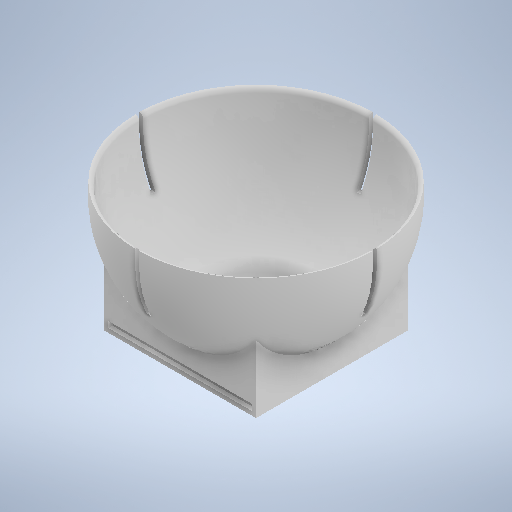
# Autodesk Inventor part: Socket
Saved by Autodesk Inventor 2025 (Build 290162000, 162)
## iProperties
Created: 2024-11-17
Part Number: Socket
Material: Generic
Document SubType Name: Modeling
Designer: ethan
Density: 1 g/cm^3
Appearance: Default
Author: ethan
Autodesk Inventor part; units mm, degrees
ref_plane "YZ Plane" through (0, 0, 0) normal (1, 0, 0) x (0, 1, 0)
sketch "Sketch1" plane through (0, 0, 0) normal (0, 0, 1) x (1, 0, 0)
  circle A0 centre (0, 0) radius 28 construction
  circle A1 centre (0, 0) radius 29 construction
  circle A2 centre (0, 0) radius 28
  circle A3 centre (0, 0) radius 29
  line L0 (0, 0) -> (27.8935, 2.4404)
  line L1 (0, 0) -> (28, 0) construction
  line L2 (0, 0) -> (0, -29.5121)
  line L3 (0, -28) -> (0, -29)
  line L4 (27.8935, 2.4404) -> (28.8971, 2.4404)
  dimension "d0" = 56
  dimension "d1" = 58
  dimension "d2" = 5
  constraints: 10 end point, 4 centre point, 4 coincident, 4 point on circle, 2 concentric, 2 horizontal, 2 point on line, 1 equal length, 1 vertical
  measures "d0" diameter of A0
  measures "d1" diameter of A1
  measures "d2" angle of L1 L0
revolve "Revolution1" add sketch "Sketch1" angle 360 about axis through (0, 0, 0) along (0, -1, 0) picked at (16.0405, -23.5642) contours A2 L4 A3 L2
sketch "Sketch2" plane through (0, 2.4404, 0) normal (0, 1, 0) x (1, 0, 0)
  line L0 (-0.5, -30) -> (0.5, -30)
  line L1 (0.5, -30) -> (0.5, 30)
  line L2 (0.5, 30) -> (-0.5, 30)
  line L3 (-0.5, 30) -> (-0.5, -30)
  line L4 (-0.5, -30) -> (0.5, 30) construction
  line L5 (0.5, -30) -> (-0.5, 30) construction
  line L6 (30, -0.5) -> (-30, -0.5)
  line L7 (-30, -0.5) -> (-30, 0.5)
  line L8 (-30, 0.5) -> (30, 0.5)
  line L9 (30, 0.5) -> (30, -0.5)
  circle A0 centre (0, 0) radius 28.8971 projected
  line L10 (30, -0.5) -> (-30, 0.5) construction
  line L11 (-30, -0.5) -> (30, 0.5) construction
  point P0 (0.5, 0.5)
  point P1 (-0.5, 0.5)
  point P2 (-0.5, -0.5)
  point P3 (0.5, -0.5)
  dimension "d4" = 1
  dimension "d5" = 60
  dimension "d6" = 60
  dimension "d7" = 1
  constraints: 24 end point, 4 midpoint, 4 parallel, 2 horizontal, 2 perpendicular
  measures "d4" distance of L2.end L1.end
  measures "d5" distance of L1.end L0.end
  measures "d6" distance of L7.end L8.end
  measures "d7" distance of L6.end L7.end
extrude "Extrusion1" cut sketch "Sketch2" against normal blind 15 contours L3 A0 L1 L0 | L3 L6 L1 A0 | L6 A0 L8 L3 | L3 L8 L1 L6 | L6 L7 L8 A0 | L1 L8 A0 L6 | A0 L8 L9 L6 | L3 A0 L1 L8 | L3 L2 L1 A0
ref_plane "Work Plane1" through (0, -29, 0) normal (0, 1, 0) x (-1, 0, 0)
sketch "Sketch3" plane through (0, -29, 0) normal (0, 1, 0) x (-1, 0, 0)
  arc A0 (-0.5, 28.8928) -> (-28.8928, 0.5) centre (0, 0) ccw projected
  arc A1 (-0.5, -26.1344) -> (0.5, -26.1344) centre (0, 0) ccw projected
  line L0 (0.5, -25.0201) -> (0.5, -26.1344) projected
  arc A2 (-0.5, -25.0201) -> (0.5, -25.0201) centre (0, 0) ccw projected
  line L1 (-0.5, -26.1344) -> (-0.5, -25.0201) projected
  circle A3 centre (0, 0) radius 26.1392
  line L2 (18.485, 18.4813) -> (-18.485, 18.4813)
  line L3 (-18.485, 18.4813) -> (-18.485, -18.4813)
  line L4 (-18.485, -18.4813) -> (18.485, -18.4813)
  line L5 (18.485, -18.4813) -> (18.485, 18.4813)
  line L6 (18.485, 18.4813) -> (-18.485, -18.4813) construction
  line L7 (-18.485, 18.4813) -> (18.485, -18.4813) construction
  dimension "d11" = 36.97
  constraints: 12 end point, 2 midpoint, 2 parallel, 2 point on circle, 1 centre point, 1 coincident, 1 horizontal, 1 perpendicular
  measures "d11" distance of L4.end L3.end
extrude "Extrusion2" add sketch "Sketch3" along normal up to surface contours L3 L2 L5 L4
sketch "Sketch4" plane through (0, -29, 0) normal (0, -1, 0) x (1, 0, 0)
  circle A0 centre (0, 0) radius 13.5
  dimension "d14" = 27
  constraints: 1 centre point, 1 coincident
  measures "d14" diameter of A0
extrude "Extrusion3" cut sketch "Sketch4" against normal blind 10
fillet "Fillet1" radius 3 1 edges at (-13.5, -24.5306, 0)
fillet "Fillet2" radius 1 4 edges at (-19.7236, 2.4404, 19.7236) (-19.7236, 2.4404, -19.7236) (19.7236, 2.4404, -19.7236) (19.7236, 2.4404, 19.7236)
sketch "Sketch5" plane through (-18.485, -29, 18.4813) normal (0, 0, 1) x (1, 0, 0)
  line L0 (0, 0) -> (0, 16.4404) construction
  line L1 (0, 0) -> (1, 0) construction
  line L2 (1, 0) -> (1, 1) construction
  line L3 (1, 1) -> (0, 1) construction
  line L4 (0, 1) -> (0, 0) construction
  arc A0 (0, 16.4404) -> (36.97, 16.4404) centre (18.485, 29) ccw construction
  line L5 (0, 0) -> (0, 16.4404) construction
  line L6 (0, 0) -> (36.97, 0) construction
  line L7 (36.97, 0) -> (36.97, 16.4404) construction
  line L8 (1, 1) -> (35.97, 1) construction
  line L9 (35.97, 1) -> (35.97, 2.5) construction
  line L10 (35.97, 2.5) -> (1, 2.5) construction
  line L11 (1, 2.5) -> (1, 1) construction
  line L12 (1, 1) -> (35.97, 1)
  line L13 (35.97, 1) -> (35.97, 2.5)
  line L14 (35.97, 2.5) -> (1, 2.5)
  line L15 (1, 2.5) -> (1, 1)
  dimension "d19" = 1
  dimension "d20" = 1
  dimension "d21" = 34.97
  dimension "d22" = 1.5
  constraints: 24 end point, 6 parallel, 3 horizontal, 3 perpendicular
  measures "d19" distance of L3.end L2.end
  measures "d20" distance of L2.end L1.end
  measures "d21" distance of L10.end L9.end
  measures "d22" distance of L9.end L8.end
extrude "Extrusion4" cut sketch "Sketch5" against normal blind 1
ref_plane "Work Plane2" through (-18.485, -29, 0) normal (0, 0, 1) x (1, 0, 0)
mirror "Mirror1" about plane through (-18.485, -29, 0) normal (0, 0, 1) of "Extrusion4"
body "Solid1"
